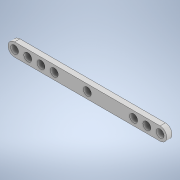
# Autodesk Inventor part: 10cmlinks
Saved by Autodesk Inventor 2022 (Build 260153000, 153)
## iProperties
Created: 2023-07-13
Part Number: 10cmlinks
Material: Generic
Document SubType Name: Modeling
Designer: jyoti
Density: 1 g/cm^3
Appearance: Default
Author: jyoti
Autodesk Inventor part; units mm, degrees
ref_plane "YZ Plane" through (0, 0, 0) normal (1, 0, 0) x (0, 1, 0)
ref_plane "XZ Plane" through (0, 0, 0) normal (0, 1, 0) x (-1, 0, 0)
ref_plane "XY Plane" through (0, 0, 0) normal (0, 0, 1) x (1, 0, 0)
sketch "Sketch1" plane through (0, 0, 0) normal (0, 0, 1) x (1, 0, 0)
  line L0 (0, 0) -> (110, 0) construction
  line L1 (0, -5) -> (110, -5)
  line L2 (110, 5) -> (0, 5)
  arc A0 (0, 5) -> (0, -5) centre (0, 0) ccw
  arc A1 (110, -5) -> (110, 5) centre (110, 0) ccw
  circle A2 centre (0, 0) radius 3
  circle A3 centre (110, 0) radius 3
  circle A4 centre (10, 0) radius 3
  circle A5 centre (100, 0) radius 3
  circle A6 centre (55, 0) radius 3
  circle A7 centre (20, 0) radius 3
  circle A8 centre (30, 0) radius 3
  circle A9 centre (90, 0) radius 3
  dimension "d0" = 110
  dimension "d1" = 10
  dimension "d2" = 6
  dimension "d3" = 6
  dimension "d4" = 6
  dimension "d5" = 6
  dimension "d6" = 6
  dimension "d7" = 6
  dimension "d8" = 6
  dimension "d9" = 6
  constraints: 10 centre point, 8 end point, 5 point on line, 4 point on circle, 4 tangent, 3 coincident, 1 horizontal, 1 midpoint, 1 parallel
  measures "d0" distance of L0.start L0.end
  measures "d1" diameter of A1
  measures "d2" diameter of A2
  measures "d3" diameter of A3
  measures "d4" diameter of A4
  measures "d5" diameter of A5
  measures "d6" diameter of A6
  measures "d7" diameter of A7
  measures "d8" diameter of A8
  measures "d9" diameter of A9
extrude "Extrusion1" add sketch "Sketch1" along normal blind 4
body "Solid1"
